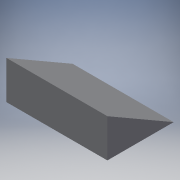
# Autodesk Inventor part: coneTela
Saved by Autodesk Inventor 2016 (Build 200138000, 138)
## iProperties
Created: 2017-06-05
Part Number: coneTela
Material: Genérico
Document SubType Name: Modeling
Designer: Fabio
Density: 1 g/cm^3
Appearance: Padrão
Author: Fabio
Autodesk Inventor part; units mm, degrees
ref_plane "YZ Plane" through (0, 0, 0) normal (1, 0, 0) x (0, 1, 0)
ref_plane "XZ Plane" through (0, 0, 0) normal (0, 1, 0) x (-1, 0, 0)
ref_plane "XY Plane" through (0, 0, 0) normal (0, 0, 1) x (1, 0, 0)
sketch "Esboço1" plane through (0, 0, 0) normal (1, 0, 0) x (0, 1, 0)
  line L0 (157.667, -62.5) -> (-58.8394, 62.5)
  line L1 (-58.8394, 62.5) -> (-58.8394, -62.5)
  line L2 (-58.8394, -62.5) -> (157.667, -62.5)
  point P0 (0, 0)
  point P1 (-58.8394, 0)
  dimension "d0" = 250
  dimension "d1" = 30
  dimension "d2" = 125
  dimension "d3" = 216.5063
  constraints: 6 end point, 1 horizontal alignment, 1 midpoint, 1 perpendicular, 1 vertical
  measures "d0" distance of L0.start L0.end
  measures "d1" angle of L2 L0
  measures "d2" distance from line of L0.end L2
  measures "d3" distance from line of L1 L0.start
extrude "Extrusão1" add sketch "Esboço1" along normal blind 330
